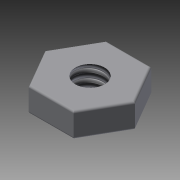
# Autodesk Inventor part: Design A Part Challenge
Saved by Autodesk Inventor 2015 (Build 190159000, 159)
## iProperties
Created: 2018-12-07
Part Number: Design A Part Challenge
Material: Generic
Document SubType Name: Modeling
Designer: 579494
Density: 1 g/cm^3
Appearance: Default
Author: 579494
Autodesk Inventor part; units mm, degrees
ref_plane "YZ Plane" through (0, 0, 0) normal (1, 0, 0) x (0, 1, 0)
ref_plane "XZ Plane" through (0, 0, 0) normal (0, 1, 0) x (-1, 0, 0)
ref_plane "XY Plane" through (0, 0, 0) normal (0, 0, 1) x (1, 0, 0)
sketch "Sketch1" plane through (0, 0, 0) normal (0, 0, 1) x (1, 0, 0)
  line L0 (0.2301, 0.4005) -> (0.4619, 0.001)
  line L1 (0.4619, 0.001) -> (0.2318, -0.3995)
  line L2 (0.2318, -0.3995) -> (-0.2301, -0.4005)
  line L3 (-0.2301, -0.4005) -> (-0.4619, -0.001)
  line L4 (-0.4619, -0.001) -> (-0.2318, 0.3995)
  line L5 (-0.2318, 0.3995) -> (0.2301, 0.4005)
  circle A0 centre (0, 0) radius 0.15
  dimension "d0" = 0.8
  dimension "d1" = 0.3
  constraints: 12 end point, 2 coincident, 1 centre point, 13 other
  measures "d0" distance between parallel lines of L2 L5
  measures "d1" diameter of A0
extrude "Extrusion1" add sketch "Sketch1" along normal blind 0.25
fillet "Fillet1" radius 0.02 12 edges at (-0.0009, 0.4, 0.25) (0.346, 0.2008, 0.25) (0.346, 0.2008, 0) (-0.0009, 0.4, 0) (0.3469, -0.1992, 0.25) (0.3469, -0.1992, 0) (0.0009, -0.4, 0) (0.0009, -0.4, 0.25) (-0.346, -0.2008, 0.25) (-0.346, -0.2008, 0) (-0.3469, 0.1992, 0.25) (-0.3469, 0.1992, 0)
thread "Thread1" size "35-282 UNM" class "2B" standard "ANSI Unified Screw Threads" full length
body "Solid1"
